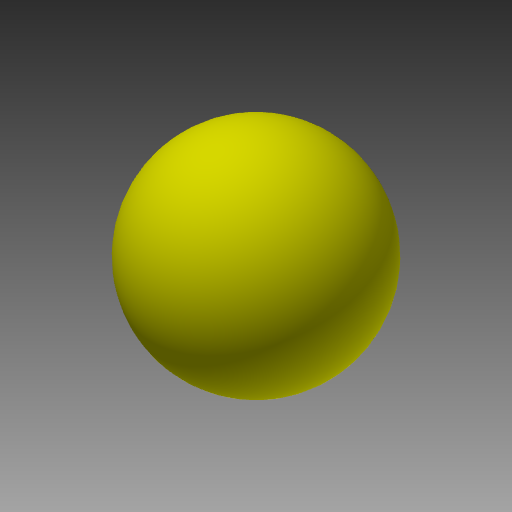
# Autodesk Inventor part: W 617/3_PART3
Saved by Autodesk Inventor 2019.1 (Build 231200000, 200)
## iProperties
Category: PARTsolutions
Company: SKF
Created: 2018-11-24
Part Number: W 617/3_PART3
Material: Allgemein
Catalog Web Link: www.cadenas.de
Description: -Deep groove ball bearings
Vendor: SKF
Document SubType Name: Modeling
Designer: psadmin
Manufacturer: SKF
Mass: 0.000268083 g
Surface Area: 0.0201062 cm^2
Volume: 0.000268083 cm^3
Density: 1 g/cm^3
Appearance: PSOLRGB-192-192-192
PSOL_IDENT_0: {$CADENAS_DATA\23d-libs\skf\bearings_units_and_housings\ball_bearings\deep_groove_ball_bearings\bb1_
PSOL_IDENT_1: 001_101.prj},193 {VTYP=3D},{NB=W 617/3_PART3},{LINA=W 617/3_PART3},{NN=BB1_001_101_PART3},{NOPRJ=TRU
PSOL_IDENT_2: E},{DATE=05.11.2018 07:58:23},{GEOMDATE=08.08.2018 12:16:40},{VERSION=},{LINEID=18990},{WBVAR=},{WBN
PSOL_IDENT_3: UMERIC=}  {NB=W 617/3_PART3},{LINA=W 617/3_PART3},{KT=DUMMY},{PRODUCTID=},{DESIGNATION=W 617/3},{DD=
PSOL_IDENT_4: 3.00},{D=6.000},{B=2.000},{C=0.000},{DD1=3.70},{DD2=0.0},{D1=4.90},{D2=0.00},{D3=0.00},{D4=0.000},{H
PSOL_IDENT_5: H=MIN},{BB=0.000},{FF=0.00},{R0MAX=MIN},{R0=MIN},{R12=0.10},{PITCH=4.30},{DW=0.800},{DDAMIN=3.600},{
PSOL_IDENT_6: DDAMAX=MIN},{DDBMIN=MIN},{DDBMAX=MIN},{DBMIN=MIN},{DAMAX=5.200},{BBAMIN=MIN},{CAMAX=MIN},{RAMAX=0.10
PSOL_IDENT_7: 0},{LOAD1=0.117},{LOAD2=0.036},{LOAD3=0.002},{SPEED1=170000},{SPEED2=110000},{KR=0.015},{F0=7.100},{
PSOL_IDENT_8: Z=8},{II=1},{MASS=0.000},{BEARING=W 617/3},{RING=},{HELP=0.550},{HELP2=0.550},{DD1ALG=1.850},{YALG=1
PSOL_IDENT_9: .850},{PITCH1=4.300},{DW1=0.800},{YALG1=2.450},{HALG1=0.550},{SH=1.850},{CU=0.240},{DESIGN=dgbbw},{H
PSOL_IDENT_10: ALG=0.35},{B1=0},{ALGO=1.000}
NT: Deep groove ball bearings
NB: W 617/3_PART3
NBSYN: $DESIGNATION._PART3
LINA: W 617/3_PART3
SUPPLIER: SKF
ARTICLENO: W 617/3_PART3
BOMINFO: W 617/3_PART3
CREATOR: CADENAS GmbH
Title: W 617/3_PART3
Author: Cadenas PARTsolutions
Comments: Deep groove ball bearings
Autodesk Inventor part; units mm, degrees
ref_plane "YZ Plane" through (0, 0, 0) normal (1, 0, 0) x (0, 1, 0)
ref_plane "XZ Plane" through (0, 0, 0) normal (0, 1, 0) x (-1, 0, 0)
ref_plane "XY Plane" through (0, 0, 0) normal (0, 0, 1) x (1, 0, 0)
sketch "Sketch_6" plane through (0, 0, 0) normal (0, 0, 1) x (1, 0, 0)
  line L0 (1.4, 2.15) -> (0.6, 2.15)
  arc A0 (1.4, 2.15) -> (0.6, 2.15) centre (1, 2.15) ccw
  line L1 (1.4, 2.15) -> (0.6, 2.15)
  dimension "d0" = 360
  constraints: 4 end point, 2 point on circle, 1 centre point
revolve "Revolution1" add sketch "Sketch_6" angle 360 about axis through (1.4, 2.15, 0) along (1, 0, 0)
body "Solid1"
